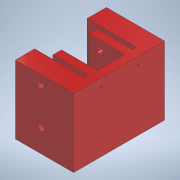
# Autodesk Inventor part: Intake Mounting Block
Saved by Autodesk Inventor 2022 (Build 260153000, 153)
## iProperties
Created: 2022-09-21
Part Number: Intake Mounting Block
Material: Generic
Document SubType Name: Modeling
Designer: matt
Density: 1 g/cm^3
Appearance: Default
Author: matt
Autodesk Inventor part; units mm, degrees
ref_plane "YZ Plane" through (0, 0, 0) normal (1, 0, 0) x (0, 1, 0)
ref_plane "XZ Plane" through (0, 0, 0) normal (0, 1, 0) x (-1, 0, 0)
ref_plane "XY Plane" through (0, 0, 0) normal (0, 0, 1) x (1, 0, 0)
sketch "Sketch2" plane through (0, 0, 0) normal (0, 1, 0) x (-1, 0, 0)
  line L0 (0, 0) -> (-48, 0)
  line L1 (-48, 0) -> (-48, -79.835)
  line L2 (-48, -79.835) -> (0, -79.835)
  line L3 (-40, -59.9175) -> (-9, -59.9175)
  line L4 (-9, -59.9175) -> (-9, -19.9175)
  line L5 (-9, -19.9175) -> (-40, -19.9175)
  line L6 (-33.9858, -17.4175) -> (3.086, -17.4175)
  line L7 (3.086, -62.4175) -> (-40, -62.4175)
  line L8 (-48, -6) -> (-48, -3.5)
  line L9 (-33.9858, -17.4175) -> (-40, -17.4175)
  line L10 (-40, -62.4175) -> (-40, -59.9175)
  line L11 (-40, -19.9175) -> (-40, -17.4175)
  line L12 (3.086, -16.9175) -> (-40.5, -16.9175)
  line L13 (-40.5, -16.9175) -> (-40.5, -20.4175)
  line L14 (-40.5, -20.4175) -> (-9.5, -20.4175)
  line L15 (-9.5, -20.4175) -> (-9.5, -59.4175)
  line L16 (-9.5, -59.4175) -> (-40.5, -59.4175)
  line L17 (-40.5, -59.4175) -> (-40.5, -62.9175)
  line L18 (-40.5, -62.9175) -> (3.086, -62.9175)
  line L19 (5, -12.8942) -> (5, -16.38) projected
  line L20 (0, 0) -> (3.086, 0)
  line L21 (3.086, 0) -> (3.086, -79.835)
  line L22 (3.086, -79.835) -> (0, -79.835)
  line L23 (3.086, -62.9175) -> (3.086, -62.4175)
  line L24 (3.086, -17.4175) -> (3.086, -16.9175)
  line L25 (3.086, -62.9175) -> (3.086, -62.4175)
  line L26 (3.086, -17.4175) -> (3.086, -16.9175)
  line L27 (-9.5, -27.9375) -> (-40.5, -27.9375)
  line L28 (-40.5, -27.9375) -> (-40.5, -51.8975)
  line L29 (-40.5, -51.8975) -> (-9.5, -51.8975)
  line L30 (-9.5, -51.8975) -> (-9.5, -27.9375)
  point P0 (-9.7436, -6)
  point P1 (0, -79.835)
  point P2 (-9.5, -51.8975)
  dimension "d19" = 79.835
  dimension "d20" = 45
  dimension "d21" = 17.4175
  dimension "d22" = 2.5
  dimension "d23" = 40
  dimension "d24" = 39
  dimension "d26" = 0.5
  dimension "d32" = 7.52
  dimension "d33" = 7.52
  dimension "d34" = 23.96
  dimension "d35" = 51.086
  constraints: 58 end point, 6 collinear, 6 parallel, 5 point on line, 4 horizontal, 3 perpendicular, 2 vertical, 7 other
  measures "d19" distance of L1.end L0.end
  measures "d20" distance between parallel lines of L7 L6
  measures "d21" distance between parallel lines of L2 L7
  measures "d24" distance between parallel lines of L4 L8
  measures "d32" distance between parallel lines of L27 L14
  measures "d33" distance between parallel lines of L16 L29
  measures "d34" distance between parallel lines of L29 L27
  measures "d35" distance between parallel lines of L1 L21
extrude "Extrusion7" add sketch "Sketch2" along normal blind 60 contours L20 L21 L12 L13 L14 L15 L27 L28 L29 L16 L17 L18 L22 L2 L1 L0
sketch "Sketch3" plane through (-3.086, 0, 0) normal (0, 0, 1) x (1, 0, 0)
  circle A0 centre (22.5, 51.8947) radius 2.8 projected
  circle A1 centre (22.5, 19.8947) radius 2.8 projected
  point P0 (3.086, 0)
  dimension "d38" = 32
  measures "d38" distance of A1.centre A0.centre
extrude "Extrusion8" cut sketch "Sketch3" against normal through all
sketch "Sketch4" plane through (-3.086, 0, -79.835) normal (-1, 0, 0) x (0, 0, 1)
  circle A0 centre (7.9375, 41) radius 2.5
  circle A1 centre (7.9375, 9) radius 2.5
  line L0 (0, 0) -> (16.9175, 0) projected
  circle A2 centre (55.9175, 52.5) radius 1.5
  circle A3 centre (23.9175, 52.5) radius 1.5
  point P0 (79.835, 0)
  dimension "d36" = 5
  dimension "d37" = 5
  dimension "d39" = 32
  dimension "d40" = 9
  dimension "d43" = 3
  constraints: 4 centre point, 1 equal radius
  measures "d36" diameter of A0
  measures "d37" diameter of A1
  measures "d39" distance of A1.centre A0.centre
  measures "d40" distance from line of L0 A1.centre
  measures "d43" diameter of A2
extrude "Extrusion9" cut sketch "Sketch4" against normal blind 20 contours A0 | A1
extrude "Extrusion10" cut sketch "Sketch4" along normal blind 10 from surface at -51.086 contours A2 | A3
equation "\"d21\" = -0.5 * d20 + 0.5 * d19"
equation "\"d33\" = d32"
body "Solid3"
